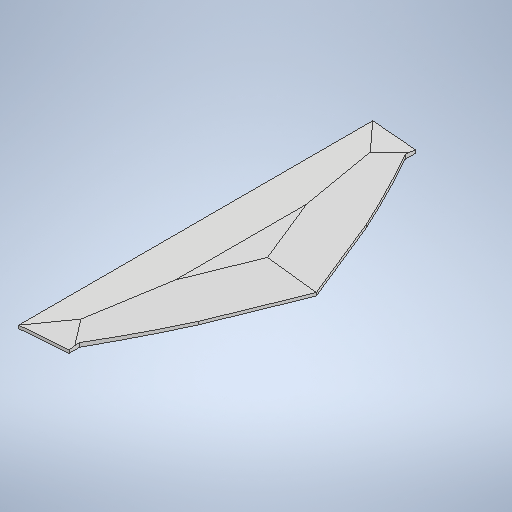
# Autodesk Inventor part: łódź
Saved by Autodesk Inventor 2025.2 (Build 292293000, 293)
## iProperties
Created: 2025-12-10
Part Number: łódź
Material: Generic
Document SubType Name: Modeling
Designer: piotr
Density: 1 g/cm^3
Appearance: Default
Author: piotr
Autodesk Inventor part; units mm, degrees
ref_plane "YZ Plane" through (0, 0, 0) normal (1, 0, 0) x (0, 1, 0)
ref_plane "XZ Plane" through (0, 0, 0) normal (0, 1, 0) x (-1, 0, 0)
ref_plane "XY Plane" through (0, 0, 0) normal (0, 0, 1) x (1, 0, 0)
sketch "Sketch1" plane through (0, 0, 0) normal (0, 1, 0) x (-1, 0, 0)
  line L0 (0, 0) -> (0, -117.5)
  line L1 (-15.4495, -1.25) -> (-15.4495, -116.25)
  line L2 (0, 0) -> (-15.4495, -1.25)
  line L3 (-15.4495, -116.25) -> (0, -117.5)
  line L4 (0, -58.75) -> (-40, -58.75)
  line L5 (-15.4495, -1.25) -> (-15.4495, -4.75)
  line L6 (-15.4495, -116.25) -> (-15.4495, -112.75)
  line L7 (-40, -58.75) -> (-28.75, -86.5607)
  line L8 (-28.75, -86.5607) -> (0, -58.75)
  arc A0 (-40, -58.75) -> (-15.4495, -112.75) centre (287.2232, 57.4375) ccw
  line L9 (0, -58.75) -> (-28.75, -30.9393)
  line L10 (-28.75, -30.9393) -> (-40, -58.75)
  arc A1 (-15.4495, -4.75) -> (-40, -58.75) centre (287.2232, -174.9375) ccw
  dimension "d0" = 117.5
  dimension "d1" = 115
  dimension "d2" = 15.5
  dimension "d3" = 15.5
  dimension "d4" = 40
  dimension "d5" = 3.5
  dimension "d6" = 3.5
  dimension "d7" = 30
  dimension "d8" = 40
  dimension "d9" = 40
  dimension "d10" = 30
  constraints: 22 end point, 6 point on circle, 2 centre point, 2 point on line, 2 vertical, 1 horizontal, 1 midpoint
  measures "d0" distance of L0.start L0.end
  measures "d1" distance of L1.start L1.end
  measures "d2" distance of L0.start L1.start
  measures "d3" distance of L1.end L0.end
  measures "d4" distance of L4.start L4.end
  measures "d5" distance of L1.start L5.end
  measures "d6" distance of L1.end L6.end
  measures "d7" distance of L4.end L7.end
  measures "d8" distance of L7.end L4.start
  measures "d9" distance of L4.start L9.end
  measures "d10" distance of L9.end L4.end
extrude "Extrusion1" add sketch "Sketch1" along normal blind 3 contours L0 L9 L1 L2 | L8 L1 L4 | L0 L3 L1 L8 | L4 L1 L9 | L4 L10 L9 L1 | L1 L8 L7 L4 | L1 A0 L8 | L9 A1 L1
chamfer "Chamfer1" distance 15 distance2 2 5 edges at (7.7248, 3, -0.625) (7.7248, 3, -116.875) (34.375, 3, -72.6554) (34.375, 3, -44.8446) (0, 3, -58.75) measured on face at (33.9115, 3, -45.0321) measured on face at (7.6844, 3, -116.3766) measured on face at (7.6844, 3, -1.1234) measured on face at (33.9115, 3, -72.4679) measured on face at (0.5, 3, -58.75)
body "Solid1"
